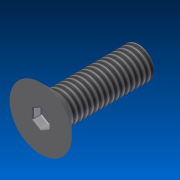
# Autodesk Inventor part: PCap(M3-8)
Saved by Autodesk Inventor 2013 (Build 170138000, 138)
## iProperties
Created: 2014-02-10
Material: 一般
Document SubType Name: Modeling
Designer: andou
Density: 1 g/cm^3
Mass: 0.0796685 g
Surface Area: 1.43734 cm^2
Volume: 0.0796685 cm^3
Author: andou
Title: PCap(M3-8)
Autodesk Inventor part; units mm, degrees
ref_plane "YZ Plane" through (0, 0, 0) normal (1, 0, 0) x (0, 1, 0)
ref_plane "XZ Plane" through (0, 0, 0) normal (0, 1, 0) x (-1, 0, 0)
ref_plane "XY Plane" through (0, 0, 0) normal (0, 0, 1) x (1, 0, 0)
sketch "スケッチ1" plane through (0, 0, 0) normal (0, 0, 1) x (1, 0, 0)
  line L0 (0, 0) -> (0, 1.5)
  line L1 (-1.5, 1.5) -> (-3, 0)
  line L2 (-3, 0) -> (0, 0)
  line L3 (-1.5, 1.5) -> (0, 1.5)
  dimension "d1" = 45
  dimension "d2" = 3
  dimension "d4" = 1.5
  constraints: 8 end point, 2 perpendicular, 1 vertical
  measures "d1" angle of L1 L2
  measures "d2" distance of L1.end L0.start
  measures "d4" distance of L1.start L0.end
revolve "回転1" add sketch "スケッチ1" angle 360 about axis through (0, 0, 0) along (0, 1, 0)
sketch "スケッチ2" plane through (0, 0, 0) normal (0, -1, 0) x (1, 0, 0)
  circle A0 centre (0, 0) radius 3 projected
  line L0 (0, 0.866) -> (0.75, 0.433)
  line L1 (0.75, 0.433) -> (0.75, -0.433)
  line L2 (0.75, -0.433) -> (0, -0.866)
  line L3 (0, -0.866) -> (-0.75, -0.433)
  line L4 (-0.75, -0.433) -> (-0.75, 0.433)
  line L5 (-0.75, 0.433) -> (0, 0.866)
  dimension "d6" = 0.75
  constraints: 12 end point, 1 coincident, 13 other
  measures "d6" distance from line of L0 point (0, 0)
extrude "押し出し1" cut sketch "スケッチ2" against normal blind 0.8 contours L0 L1 L2 L3 L4 L5
sketch "スケッチ3" plane through (0, 1.5, 0) normal (0, 1, 0) x (1, 0, 0)
  circle A0 centre (0, 0) radius 1.5 projected
extrude "押し出し2" add sketch "スケッチ3" along normal blind 8
chamfer "面取り1" distance 0.1 angle 45 7 edges at (-1.5, 9.5, 0) (-0.375, 0, -0.6495) (0.375, 0, -0.6495) (0.75, 0, 0) (0.375, 0, 0.6495) (-0.375, 0, 0.6495) (-0.75, 0, 0)
fillet "フィレット1" radius 0.1 24 edges at (0.75, 0.8, 0) (0.375, 0.8, -0.6495) (0.75, 0.45, -0.433) (0, 0.45, -0.866) (-0.375, 0.8, -0.6495) (-0.75, 0.45, -0.433) (-0.75, 0.8, 0) (-0.75, 0.45, 0.433) (-0.375, 0.8, 0.6495) (0.75, 0.45, 0.433) (0.375, 0.8, 0.6495) (0, 0.45, 0.866) (0.425, 0, -0.7361) (0.85, 0, 0) (0.425, 0, 0.7361) (-0.425, 0, 0.7361) (-0.85, 0, 0) (-0.425, 0, -0.7361) (0.8, 0.05, -0.4619) (0, 0.05, -0.9238) (0.8, 0.05, 0.4619) (0, 0.05, 0.9238) (-0.8, 0.05, 0.4619) (-0.8, 0.05, -0.4619)
thread "ねじ2" size "M3x0.5" class "6g" standard "ANSI Metric M Profile" full length
